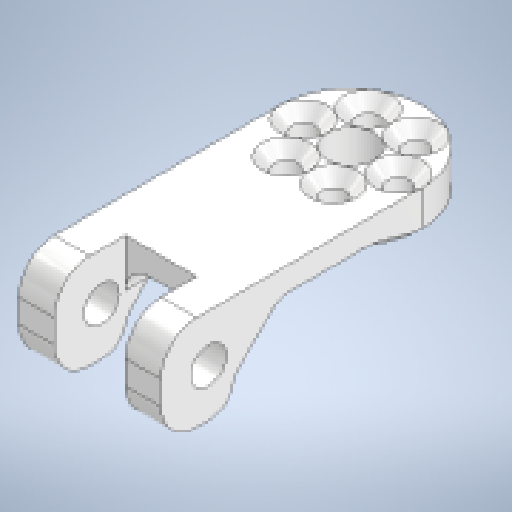
# Autodesk Inventor part: Plowette - Mount
Saved by Autodesk Inventor 2023.2 (Build 272271000, 271)
## iProperties
Created: 2023-04-05
Part Number: Plowette - Mount
Material: UHMW, White
Document SubType Name: Modeling
Designer: Nathan Cai
Density: 0.94 g/cm^3
Appearance: Smooth - White
Mass: 2.90425 g
Surface Area: 26.8531 cm^2
Volume: 3.08962 cm^3
Author: Nathan Cai
Autodesk Inventor part; units mm, degrees
ref_plane "YZ Plane" through (0, 0, 0) normal (1, 0, 0) x (0, 1, 0)
ref_plane "XZ Plane" through (0, 0, 0) normal (0, 1, 0) x (-1, 0, 0)
ref_plane "XY Plane" through (0, 0, 0) normal (0, 0, 1) x (1, 0, 0)
sketch "Sketch1" plane through (0, 0, 0) normal (0, 1, 0) x (-1, 0, 0)
  circle A0 centre (0, 0) radius 6.35 construction
  circle A1 centre (0, 0) radius 3.175
  line L0 (0, 0) -> (6.35, 0) construction
  circle A2 centre (6.35, 0) radius 1.5875
  circle A3 centre (3.175, 5.4993) radius 1.5875
  circle A4 centre (-3.175, 5.4993) radius 1.5875
  circle A5 centre (-6.35, 0) radius 1.5875
  circle A6 centre (-3.175, -5.4993) radius 1.5875
  circle A7 centre (3.175, -5.4993) radius 1.5875
  circle A8 centre (0, 0) radius 9.525
  dimension "d0" = 12.7
  dimension "d1" = 6.35
  dimension "d2" = 3.175
  dimension "d5" = 360
  dimension "d7" = 19.05
  constraints: 8 centre point, 4 coincident, 2 end point, 1 horizontal, 1 horizontal alignment, 15 other
  measures "d1" diameter of A1
  measures "d2" diameter of A2
  measures "d7" diameter of A8
extrude "Extrusion1" add sketch "Sketch1" along normal blind 1.5875
sketch "Sketch2" plane through (0, 1.5875, 0) normal (0, 1, 0) x (1, 0, 0)
  circle A0 centre (0, 0) radius 9.525 construction
  circle A1 centre (-3.175, 5.4993) radius 1.5875 projected
  circle A2 centre (3.175, 5.4993) radius 1.5875 projected
  circle A3 centre (6.35, 0) radius 1.5875 projected
  circle A4 centre (3.175, -5.4993) radius 1.5875 projected
  circle A5 centre (-3.175, -5.4993) radius 1.5875 projected
  circle A6 centre (-6.35, 0) radius 1.5875 projected
  circle A7 centre (0, 0) radius 3.175 projected
  line L0 (0, 0) -> (0, -25.4) construction
  line L1 (-9.525, 0) -> (-9.525, -25.4)
  line L2 (9.525, -25.4) -> (9.525, 0)
  arc A8 (9.525, 0) -> (-9.525, 0) centre (0, 0) ccw
  arc A9 (-9.525, -25.4) -> (9.525, -25.4) centre (0, -25.4) ccw construction
  circle A10 centre (0, 0) radius 9.525 projected
  line L3 (-9.525, -34.925) -> (9.525, -34.925)
  line L4 (9.525, -34.925) -> (9.525, -15.875)
  line L5 (9.525, -15.875) -> (-9.525, -15.875) construction
  line L6 (-9.525, -15.875) -> (-9.525, -34.925)
  line L7 (-9.525, -34.925) -> (9.525, -15.875) construction
  line L8 (9.525, -34.925) -> (-9.525, -15.875) construction
  point P0 (0, -12.7)
  dimension "d10" = 25.4
  constraints: 20 end point, 5 tangent, 4 point on circle, 3 midpoint, 3 parallel, 2 centre point, 1 horizontal, 1 perpendicular, 1 point on line, 1 vertical, 2 other
  measures "d10" distance of L0.start L0.end
extrude "Extrusion2" add sketch "Sketch2" along normal blind 3.175
fillet "Fillet1" radius 3.175 1 edges at (0, 1.5875, 9.525)
sketch "Sketch3" plane through (0, 1.5875, 0) normal (0, -1, 0) x (1, 0, 0)
  line L0 (9.525, 34.925) -> (9.525, 0) projected
  line L1 (9.525, 34.925) -> (-9.525, 34.925)
  line L2 (-9.525, 34.925) -> (-9.525, 25.4)
  line L3 (-9.525, 25.4) -> (9.525, 25.4)
  line L4 (9.525, 25.4) -> (9.525, 34.925)
  point P0 (0, 0)
  dimension "d14" = 19.05
  dimension "d15" = 9.525
  constraints: 8 end point, 2 parallel, 1 horizontal, 1 perpendicular
  measures "d14" distance of L3.end L2.end
  measures "d15" distance of L2.end L1.end
extrude "Extrusion3" add sketch "Sketch3" along normal blind 9.525
sketch "Sketch4" plane through (0, -7.9375, 0) normal (0, -1, 0) x (1, 0, 0)
  line L0 (-4.7625, 44.45) -> (4.7625, 44.45)
  line L1 (4.7625, 44.45) -> (4.7625, 25.4)
  line L2 (4.7625, 25.4) -> (-4.7625, 25.4)
  line L3 (-4.7625, 25.4) -> (-4.7625, 44.45)
  line L4 (-9.525, 34.925) -> (9.525, 34.925) projected
  line L5 (-4.7625, 44.45) -> (4.7625, 25.4) construction
  line L6 (4.7625, 44.45) -> (-4.7625, 25.4) construction
  point P0 (0, 0)
  point P1 (0, 34.925)
  dimension "d18" = 9.525
  dimension "d19" = 9.525
  constraints: 12 end point, 3 midpoint, 2 parallel, 1 horizontal, 1 perpendicular
  measures "d18" distance of L1.end L2.end
  measures "d19" distance between parallel lines of L2 L4
extrude "Extrusion4" cut sketch "Sketch4" against normal through all
chamfer "Chamfer1" distance 6.35 angle 45 2 edges at (7.1438, 1.5875, 25.4) (-7.1437, 1.5875, 25.4)
sketch "Sketch5" plane through (-9.525, 4.7625, 0) normal (-1, 0, 0) x (0, 0, 1)
  circle A0 centre (28.575, -6.35) radius 2.3813
  line L0 (34.925, -12.7) -> (34.925, 0) projected
  line L1 (34.925, -6.35) -> (19.0712, -6.35) construction
  point P0 (0, -4.7625)
  dimension "d25" = 4.7625
  dimension "d26" = 6.35
  constraints: 2 end point, 1 centre point, 1 horizontal, 1 midpoint, 1 point on line
  measures "d25" diameter of A0
  measures "d26" distance from line of L0 A0.centre
extrude "Extrusion5" cut sketch "Sketch5" against normal through all
fillet "Fillet2" radius 3.175 8 edges at (7.1437, 1.5875, 19.05) (7.1438, -4.7625, 25.4) (7.1438, -7.9375, 25.4) (-7.1438, -4.7625, 25.4) (-7.1437, -7.9375, 25.4) (-7.1438, 1.5875, 19.05) (4.7625, 1.5875, 22.225) (-4.7625, 1.5875, 22.225)
fillet "Fillet3" radius 4.7625 4 edges at (7.1438, -7.9375, 34.925) (-7.1437, -7.9375, 34.925) (7.1438, 4.7625, 34.925) (-7.1437, 4.7625, 34.925)
chamfer "Chamfer2" distance 1.5875 angle 45 6 edges at (1.5875, 4.7625, 5.4993) (-4.7625, 4.7625, 5.4993) (4.7625, 4.7625, 0) (1.5875, 4.7625, -5.4993) (-4.7625, 4.7625, -5.4993) (-7.9375, 4.7625, 0)
body "Solid1"
